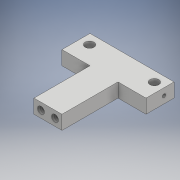
# Autodesk Inventor part: holder square
Saved by Autodesk Inventor 2017.3 (Build 213256000, 256)
## iProperties
Created: 2017-12-04
Part Number: holder square
Material: Generic
Document SubType Name: Modeling
Designer: Mac
Density: 1 g/cm^3
Appearance: Default
Author: Mac
Autodesk Inventor part; units mm, degrees
ref_plane "YZ Plane" through (0, 0, 0) normal (1, 0, 0) x (0, 1, 0)
ref_plane "XZ Plane" through (0, 0, 0) normal (0, 1, 0) x (-1, 0, 0)
ref_plane "XY Plane" through (0, 0, 0) normal (0, 0, 1) x (1, 0, 0)
sketch "Sketch1" plane through (0, 0, 0) normal (0, 0, 1) x (1, 0, 0)
  line L0 (-15, -10) -> (15, -10)
  line L1 (15, -10) -> (15, 10)
  line L2 (15, 10) -> (-15, 10)
  line L3 (-15, 10) -> (-15, -10)
  point P0 (0, 0)
  dimension "d0" = 30
  dimension "d1" = 20
  constraints: 8 end point, 2 parallel, 1 horizontal, 1 perpendicular
  measures "d0" distance of L2.end L1.end
  measures "d1" distance of L1.end L0.end
extrude "Extrusion1" add sketch "Sketch1" along normal blind 5
sketch "Sketch4" plane through (-15, -10, 0) normal (0, -1, 0) x (1, 0, 0)
  line L0 (0, 5) -> (30, 5) projected
  line L1 (0, 5) -> (30, 5)
  line L2 (30, 5) -> (30, 0)
  line L3 (30, 0) -> (0, 0)
  line L4 (0, 0) -> (0, 5)
  point P0 (15, 0)
  constraints: 8 end point, 2 parallel, 1 horizontal, 1 perpendicular
extrude "Extrusion3" cut sketch "Sketch4" against normal blind 10
sketch "Sketch5" plane through (0, 0, 5) normal (0, 0, 1) x (1, 0, 0)
  circle A0 centre (-11.579, 6.421) radius 1.5875
  circle A1 centre (11.579, 6.421) radius 1.5875
  point P0 (0, 0)
  dimension "d10" = 3.175
  dimension "d11" = 3.175
  constraints: 2 centre point
  measures "d10" diameter of A0
  measures "d11" diameter of A1
extrude "Extrusion4" cut sketch "Sketch5" against normal blind 5
sketch "Sketch6" plane through (-15, 10, 0) normal (-1, 0, 0) x (0, 0, 1)
  point P0 (0, -10)
  point P1 (2.5, -3.579)
sketch "Sketch7" plane through (15, 10, 5) normal (1, 0, 0) x (0, 0, -1)
  point P0 (5, -10)
  point P1 (2.5, -3.579)
hole "Hole2" at (-15, 6.421, 2.5) direction (1, 0, 0) diameter 1.221 depth 3 tip angle 118 thread size "M1.6x0.35" class "6H" standard "ISO Metric profile"
hole "Hole3" at (15, 6.421, 2.5) direction (-1, 0, 0) diameter 1.221 depth 3 tip angle 118 thread size "M1.6x0.35" class "6H" standard "ISO Metric profile"
sketch "Sketch9" plane through (-15, 0, 0) normal (0, -1, 0) x (1, 0, 0)
  line L0 (10, 0) -> (20, 0)
  line L1 (20, 0) -> (20, 5)
  line L2 (20, 5) -> (10, 5)
  line L3 (10, 5) -> (10, 0)
  point P0 (15, 0)
  dimension "d35" = 10
  dimension "d36" = 5
  constraints: 8 end point, 2 parallel, 1 horizontal, 1 perpendicular
  measures "d35" distance of L2.end L1.end
  measures "d36" distance of L1.end L0.end
extrude "Extrusion5" add sketch "Sketch9" along normal blind 20
sketch "Sketch10" plane through (-15, -20, 0) normal (0, -1, 0) x (1, 0, 0)
  point P0 (15, 0)
  point P1 (12.5, 2.5)
  point P2 (17.5, 2.5)
hole "Hole4" at (-2.5, -20, 2.5) at (2.5, -20, 2.5) direction (0, 1, 0) diameter 2.487 depth 10 tip angle 118 thread size "5-40 UNC" class "2B" standard "ANSI Unified Screw Threads"
body "Solid1"
